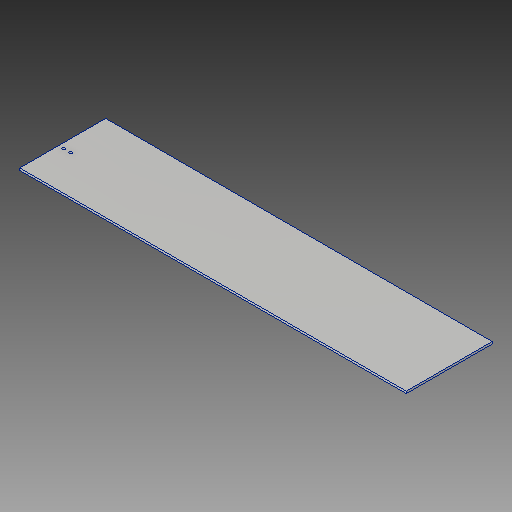
# Autodesk Inventor part: Support Sheet
Saved by Autodesk Inventor 2017 (Build 210142000, 142)
## iProperties
Created: 2018-01-26
Part Number: Support Sheet
Material: Aluminum 6061
Document SubType Name: Modeling
Designer: S346795925
Density: 2.7 g/cm^3
Appearance: Aluminum - Flat
Author: S346795925
Autodesk Inventor part; units mm, degrees
ref_plane "YZ Plane" through (0, 0, 0) normal (1, 0, 0) x (0, 1, 0)
ref_plane "XZ Plane" through (0, 0, 0) normal (0, 1, 0) x (-1, 0, 0)
ref_plane "XY Plane" through (0, 0, 0) normal (0, 0, 1) x (1, 0, 0)
sketch "Sketch1" plane through (0, 0, 0) normal (0, 1, 0) x (-1, 0, 0)
  line L0 (0, 0) -> (571.5, 0)
  line L1 (571.5, 0) -> (571.5, 127)
  line L2 (571.5, 127) -> (0, 127)
  line L3 (0, 127) -> (0, 0)
  dimension "d0" = 571.5
  dimension "d1" = 127
  constraints: 8 end point, 2 parallel, 1 horizontal, 1 perpendicular
  measures "d0" distance of L2.end L1.end
  measures "d1" distance of L1.end L0.end
extrude "Extrusion1" add sketch "Sketch1" along normal blind 3.175
sketch "Sketch2" plane through (0, 3.175, 0) normal (0, 1, 0) x (1, 0, 0)
  circle A0 centre (-563.7967, -69.9237) radius 2.25
  circle A1 centre (-553.2967, -69.9237) radius 2.2479
  point P0 (0, 0)
  dimension "d23" = 4.4958
  dimension "d24" = 10.5
  constraints: 2 centre point, 1 horizontal alignment
  measures "d23" diameter of A1
  measures "d24" distance of A0.centre A1.centre
extrude "Extrusion4" cut sketch "Sketch2" against normal through all
body "Solid1"
